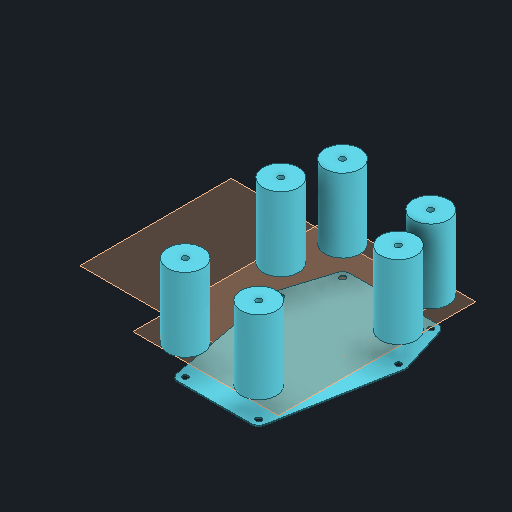
# Autodesk Inventor part: body_composition
Saved by Autodesk Inventor 2026 (Build 300175000, 175)
## iProperties
Created: 2026-04-26
Part Number: body_composition
Material: Сталь
Document SubType Name: Modeling
Designer: user
Density: 7.85 g/cm^3
Appearance: Серо-синий
Mass: 1256.55 g
Surface Area: 1105.69 cm^2
Volume: 160.07 cm^3
Author: user
Autodesk Inventor part; units mm, degrees
ref_plane "YZ Plane" through (0, 0, 0) normal (1, 0, 0) x (0, 1, 0)
ref_plane "XY Plane" through (0, 0, 0) normal (0, 0, 1) x (1, 0, 0)
ref_plane "РабПлоскость1" through (0, 500, 0) normal (0, 1, 0) x (-1, 0, 0)
sketch "Эскиз5" plane through (0, 500, 0) normal (0, 1, 0) x (-1, 0, 0)
  circle A0 centre (-150, 25) radius 10
  line L0 (0, -2.2566) -> (0, 604.845)
  circle A1 centre (-200, 185) radius 10
  circle A2 centre (-125, 585) radius 10
  arc A3 (-125, 610) -> (-149.5718, 589.6072) centre (-125, 585) ccw
  arc A4 (-224.5718, 189.6072) -> (-223.862, 177.5431) centre (-200, 185) ccw
  arc A5 (-173.862, 17.5431) -> (-150, 0) centre (-150, 25) ccw
  line L1 (-149.5718, 589.6072) -> (-224.5718, 189.6072)
  line L2 (-223.862, 177.5431) -> (-173.862, 17.5431)
  line L3 (-125, 610) -> (0, 610)
  line L4 (-150, 0) -> (0, 0)
  line L5 (223.862, 177.5431) -> (173.862, 17.5431)
  arc A6 (223.862, 177.5431) -> (224.5718, 189.6072) centre (200, 185) ccw
  circle A7 centre (200, 185) radius 10
  arc A8 (150, 0) -> (173.862, 17.5431) centre (150, 25) ccw
  circle A9 centre (150, 25) radius 10
  line L6 (150, 0) -> (0, 0)
  line L7 (149.5718, 589.6072) -> (224.5718, 189.6072)
  circle A10 centre (125, 585) radius 10
  arc A11 (149.5718, 589.6072) -> (125, 610) centre (125, 585) ccw
  line L8 (125, 610) -> (0, 610)
  dimension "d19" = 300
  dimension "d20" = 400
  dimension "d21" = 250
  dimension "d22" = 400
  dimension "d23" = 160
  dimension "d24" = 20
  dimension "d25" = 50
  constraints: 18 end point, 12 centre point, 12 point on circle, 12 symmetric about line, 7 coincident, 6 tangent, 4 equal radius, 2 perpendicular, 2 point on line, 1 vertical, 6 other
  measures "d19" diameter of A0.centre L0
  measures "d20" diameter of A1.centre L0
  measures "d21" diameter of A2.centre L0
  measures "d22" vertical distance of A1.centre A2.centre
  measures "d23" vertical distance of A1.centre A0.centre
  measures "d24" diameter of A0
  measures "d25" diameter of A3
extrude "Выдавливание5" add sketch "Эскиз5" along normal blind 3
ref_plane "РабПлоскость2" through (0, 603, 0) normal (0, 1, 0) x (1, 0, 0)
sketch "Эскиз9" plane through (0, 603, 0) normal (0, 1, 0) x (1, 0, 0)
  line L0 (150, 0) -> (-150, 0) projected
  arc A0 (-150, 0) -> (-173.862, -17.5431) centre (-150, -25) ccw projected
  line L1 (-173.862, -17.5431) -> (-223.862, -177.5431) projected
  arc A1 (-223.862, -177.5431) -> (-224.5718, -189.6072) centre (-200, -185) ccw projected
  line L2 (-224.5718, -189.6072) -> (-149.5718, -589.6072) projected
  arc A2 (-149.5718, -589.6072) -> (-125, -610) centre (-125, -585) ccw projected
  line L3 (-125, -610) -> (125, -610) projected
  arc A3 (125, -610) -> (149.5718, -589.6072) centre (125, -585) ccw projected
  line L4 (149.5718, -589.6072) -> (224.5718, -189.6072) projected
  arc A4 (224.5718, -189.6072) -> (223.862, -177.5431) centre (200, -185) ccw projected
  line L5 (223.862, -177.5431) -> (173.862, -17.5431) projected
  arc A5 (173.862, -17.5431) -> (150, 0) centre (150, -25) ccw projected
  circle A6 centre (-125, -585) radius 10 projected
  circle A7 centre (-150, -25) radius 10 projected
  circle A8 centre (-200, -185) radius 10 projected
  circle A9 centre (200, -185) radius 10 projected
  circle A10 centre (125, -585) radius 10 projected
  circle A11 centre (150, -25) radius 10 projected
  circle A12 centre (150, -25) radius 60
  circle A13 centre (-150, -25) radius 60
  circle A14 centre (-200, -185) radius 60
  circle A15 centre (200, -185) radius 60
  circle A16 centre (125, -585) radius 60
  circle A17 centre (-125, -585) radius 60
  point P0 (0, 0)
  dimension "d42" = 120
  dimension "d43" = 120
  dimension "d44" = 120
  constraints: 6 centre point, 6 coincident, 3 equal radius
  measures "d42" diameter of A12
  measures "d43" diameter of A13
  measures "d44" diameter of A14
extrude "Выдавливание6" add sketch "Эскиз9" along normal blind 250 contours A5 L5 A12 L0 | L0 A12 L5 A5 | A13 L1 A0 L0 | L0 A0 L1 A13 | A15 L4 A4 L5 | L5 A4 L4 A15 | A14 L2 A1 L1 | L1 A1 L2 A14 | A16 L3 A3 L4 | L4 A3 L3 A16 | A17 L3 A2 L2 | L2 A2 L3 A17
equation "\"d24\" = d31"
equation "\"d32\" = thickness_steel"
equation "\"tolerance_plazma\" = 0.1"
equation "\"thickness_steel\" = 3"
equation "\"d_main_screw_holes\" = 6.1"
equation "\"d_main_shaft\" = 15"
equation "\"thickness_profile_tibea\" = 3"
equation "\"hight_shaft_shift\" = 37"
equation "\"thickness_profile_femur\" = 3"
equation "\"width_shaft_shift\" = 35"
equation "\"width_flattened_surface\" = 12"
equation "\"d31\" = 20"
